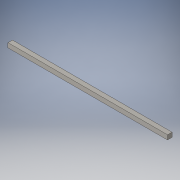
# Autodesk Inventor part: Drum_Key
Saved by Autodesk Inventor 2016 (Build 200138000, 138)
## iProperties
Created: 2016-03-01
Part Number: Drum_Key
Material: Steel, Carbon
Document SubType Name: Modeling
Designer: agmle
Mass: 9.54739 g
Surface Area: 15.5242 cm^2
Volume: 1.21623 cm^3
Density: 7.85 g/cm^3
Appearance: Semi-Polished
Author: agmle
Autodesk Inventor part; units mm, degrees
ref_plane "YZ Plane" through (0, 0, 0) normal (1, 0, 0) x (0, 1, 0)
ref_plane "XZ Plane" through (0, 0, 0) normal (0, 1, 0) x (-1, 0, 0)
ref_plane "XY Plane" through (0, 0, 0) normal (0, 0, 1) x (1, 0, 0)
sketch "Sketch1" plane through (0, 0, 0) normal (1, 0, 0) x (0, 1, 0)
  line L0 (1.5875, 1.5875) -> (-1.5875, 1.5875)
  line L1 (-1.5875, 1.5875) -> (-1.5875, -1.5875)
  line L2 (-1.5875, -1.5875) -> (1.5875, -1.5875)
  line L3 (1.5875, -1.5875) -> (1.5875, 1.5875)
  line L4 (0, 1.5875) -> (0, -1.5875) construction
  point P0 (0, 0)
  point P1 (0, 0)
  dimension "d0" = 3.175
  dimension "d1" = 3.175
  constraints: 10 end point, 3 midpoint, 2 parallel, 1 coincident, 1 horizontal, 1 perpendicular
  measures "d0" distance of L2.end L0.start
  measures "d1" distance of L0.start L0.end
extrude "Extrusion1" add sketch "Sketch1" along normal blind 112.776
equation "\"d0\" = Gearbox_Shaft_Key_Width"
equation "\"d1\" = Gearbox_Shaft_Key_Height"
equation "\"Gearbox_Shaft_OD\" = 12.7"
equation "\"Gearbox_Shaft_Key_Width\" = 3.175"
equation "\"Gearbox_Shaft_Key_Height\" = 3.175"
equation "\"Drum_Spool_OD\" = 50.8"
equation "\"Drum_Wall_OD\" = 76.2"
equation "\"Drum_Spool_Width\" = 50.8"
equation "\"Drum_Wall_Width\" = 6.35"
equation "\"Break_Edge\" = 1"
equation "\"Fitting_Break\" = 2"
body "Solid1"
